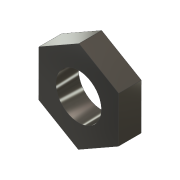
# Autodesk Inventor part: hex
Saved by Autodesk Inventor 2016 (Build 200138000, 138)
## iProperties
Created: 2020-10-21
Part Number: hex
Material: Generic
Document SubType Name: Modeling
Designer: extract
Density: 1 g/cm^3
Appearance: Default
Author: extract
Autodesk Inventor part; units mm, degrees
ref_plane "YZ Plane" through (0, 0, 0) normal (1, 0, 0) x (0, 1, 0)
ref_plane "XZ Plane" through (0, 0, 0) normal (0, 1, 0) x (-1, 0, 0)
ref_plane "XY Plane" through (0, 0, 0) normal (0, 0, 1) x (1, 0, 0)
sketch "Sketch1" plane through (0, 0, 0) normal (0, 1, 0) x (-1, 0, 0)
  circle A0 centre (0, 0) radius 2
  line L0 (3.5123, -2) -> (0.0241, -4.0418)
  line L1 (0.0241, -4.0418) -> (-3.4882, -2.0418)
  line L2 (-3.4882, -2.0418) -> (-3.5123, 2)
  line L3 (-3.5123, 2) -> (-0.0241, 4.0418)
  line L4 (-0.0241, 4.0418) -> (3.4882, 2.0418)
  line L5 (3.4882, 2.0418) -> (3.5123, -2)
  dimension "d0" = 4
  constraints: 12 end point, 2 coincident, 1 centre point, 13 other
  measures "d0" diameter of A0
extrude "Extrusion1" add sketch "Sketch1" along normal blind 2
body "Solid1"
